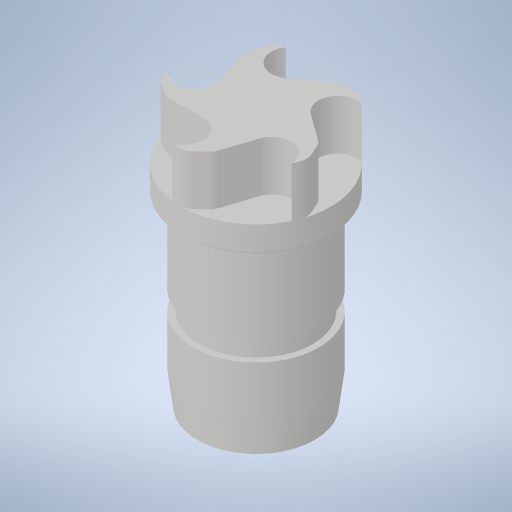
# Autodesk Inventor part: 3.2mm_uncorrected_thin
Saved by Autodesk Inventor 2023.1 (Build 271208000, 208)
## iProperties
Created: 2020-02-22
Part Number: 3.2mm_uncorrected_thin
Material: Generic
Document SubType Name: Modeling
Designer: kongooi
Density: 1 g/cm^3
Appearance: Default
Author: kongooi
Autodesk Inventor part; units mm, degrees
ref_plane "YZ Plane" through (0, 0, 0) normal (1, 0, 0) x (0, 1, 0)
sketch "Sketch2" plane through (0, 0, 0) normal (0, 1, 0) x (-1, 0, 0)
  line L0 (-0.3288, 1.3184) -> (-0.1582, 1.472)
  line L1 (-0.3288, 1.3184) -> (-0.1582, 1.472)
  line L2 (-0.5094, -1.2599) -> (-0.7376, -1.2837)
  arc A0 (0.7438, -1.3598) -> (0.1795, -0.809) centre (0.4146, -1.1327) ccw
  line L3 (-0.365, -1.2045) -> (0.1795, -0.809)
  arc A1 (-1.0634, -1.1277) -> (-0.954, -1.2216) centre (-0.0001, 0.0001) ccw
  line L4 (-0.365, -1.2045) -> (0.1795, -0.809)
  arc A2 (-0.5094, -1.2599) -> (-0.365, -1.2045) centre (-0.5404, -0.963) ccw
  line L5 (1.1525, 0.72) -> (1.3512, 0.6052)
  arc A3 (0.1974, 1.5374) -> (0.3303, 0.7602) centre (0.3304, 1.1602) ccw
  line L6 (1.0031, 0.7601) -> (0.3303, 0.7602)
  arc A4 (1.1525, 0.72) -> (1.0031, 0.7601) centre (1.0031, 0.4616) ccw
  line L7 (1.0407, -0.8744) -> (0.993, -1.0981)
  arc A5 (1.5231, 0.2873) -> (0.8243, -0.0783) centre (1.2047, 0.0452) ccw
  line L8 (1.0326, -0.7199) -> (0.8243, -0.0783)
  arc A6 (1.0407, -0.8744) -> (1.0326, -0.7199) centre (0.7487, -0.8121) ccw
  arc A7 (-1.4012, 0.663) -> (-0.621, 0.5492) centre (-1.0013, 0.6728) ccw
  line L9 (-0.413, 1.1889) -> (-0.621, 0.5492)
  arc A8 (-0.3288, 1.3184) -> (-0.413, 1.1889) centre (-0.1291, 1.0966) ccw
  line L10 (-1.3557, 0.0951) -> (-1.4489, 0.3047)
  arc A9 (-1.0634, -1.1277) -> (-0.7141, -0.4208) centre (-0.9492, -0.7444) ccw
  line L11 (-1.2585, -0.0252) -> (-0.7141, -0.4208)
  arc A10 (-1.3557, 0.0951) -> (-1.2585, -0.0252) centre (-1.083, 0.2163) ccw
  arc A11 (1.5231, 0.2872) -> (1.4898, 0.4277) centre (-0.0001, 0.0001) ccw
  arc A12 (-1.4012, 0.663) -> (-1.4567, 0.5298) centre (-0.0001, 0.0001) ccw
  arc A13 (0.7438, -1.3598) -> (0.867, -1.2847) centre (-0.0001, 0.0001) ccw
  arc A14 (0.1974, 1.5374) -> (0.0535, 1.5491) centre (-0.0001, 0.0001) ccw
  arc A15 (0.0535, 1.5491) -> (-0.1582, 1.472) centre (0.0431, 1.2484) ccw
  arc A16 (-1.4567, 0.5298) -> (-1.4489, 0.3047) centre (-1.174, 0.4269) ccw
  arc A17 (1.4898, 0.4277) -> (1.3512, 0.6052) centre (1.2005, 0.3447) ccw
  arc A18 (-0.954, -1.2216) -> (-0.7376, -1.2837) centre (-0.7688, -0.9844) ccw
  arc A19 (0.867, -1.2847) -> (0.993, -1.0981) centre (0.6987, -1.0353) ccw
  circle A20 centre (-0.0001, 0.0001) radius 1.55
  point P0 (-1.356, 0.0956)
  point P1 (1.0033, 0.76)
  point P2 (0.3301, 0.76)
  dimension "d305" = 3.1
  constraints: 49 point on circle, 26 tangent, 24 end point, 20 centre point, 12 equal radius, 2 coincident, 2 collinear, 3 other
sketch "Sketch3" plane through (0, 0, 0) normal (0, 1, 0) x (-1, 0, 0)
  line L0 (5.0133, 39.043) -> (38.6813, 7.297)
  line L1 (38.6813, 7.297) -> (18.893, -34.5332)
  line L2 (18.893, -34.5332) -> (-27.0048, -28.6397)
  line L3 (-27.0048, -28.6397) -> (-35.5829, 16.8329)
  line L4 (-35.5829, 16.8329) -> (5.0133, 39.043)
  circle A0 centre (0, 0) radius 39.3635
  circle A1 centre (0, 0) radius 20.4353
  circle A2 centre (0, 0) radius 31.8458
  circle A3 centre (10.4717, -28.7325) radius 10.093
  circle A4 centre (41.1153, -0.5956) radius 4.0726
  circle A5 centre (8.144, 29.3283) radius 10.0252
  circle A6 centre (-25.3778, 16.9956) radius 10.0583
  circle A7 centre (-24.1576, -18.872) radius 10.1582
  line L5 (-25.3778, 16.9956) -> (8.3216, 29.3877)
  line L6 (8.3216, 29.3877) -> (30.5209, 1.1669)
  line L7 (30.5209, 1.1669) -> (10.5413, -28.6665)
  line L8 (10.5413, -28.6665) -> (-24.006, -18.8838)
  line L9 (-24.006, -18.8838) -> (-25.3778, 16.9956)
  line L10 (-31.306, -23.8626) -> (-32.3687, 22.3998)
  line L11 (-32.3687, 22.3998) -> (11.301, 37.7064)
  line L12 (11.301, 37.7064) -> (39.3531, 0.904)
  line L13 (39.3531, 0.904) -> (13.0206, -37.1477)
  line L14 (13.0206, -37.1477) -> (-31.306, -23.8626)
  point P0 (-9.1427, -30.5051)
  constraints: 30 end point, 6 centre point, 6 coincident, 4 tangent, 1 midpoint, 43 other
extrude "Extrusion4" add sketch "Sketch2" against normal blind 1.032 contours L0 A15 A14 A3 L6 A4 L5 A17 A11 A5 L8 A6 L7 A19 A13 A0 L3 A2 L2 A18 A1 A9 L11 A10 L10 A16 A12 A7 L9 A8
sketch "Sketch6" plane through (0, -1.032, 0) normal (0, -1, 0) x (1, 0, 0)
  circle A0 centre (0, 0) radius 1.55
  dimension "d304" = 3.1
  constraints: 1 centre point, 1 coincident
  measures "d304" diameter of A0
extrude "Extrusion5" add sketch "Sketch6" along normal blind 0.55
ref_plane "Plan de construction1" through (0, -1.582, 0) normal (0, -1, 0) x (1, 0, 0)
sketch "Sketch7" plane through (0, -1.582, 0) normal (0, -1, 0) x (1, 0, 0)
  circle A0 centre (0, 0) radius 1.3
  circle A1 centre (0, 0) radius 0.6
  circle A2 centre (0, 0) radius 1.175
  dimension "d303" = 2.6
  dimension "d306" = 1.2
  dimension "d307" = 2.35
  constraints: 3 centre point, 2 coincident
  measures "d303" diameter of A0
  measures "d306" diameter of A1
  measures "d307" diameter of A2
extrude "Extrusion6" add sketch "Sketch7" along normal blind 3.8 contours A0 | A2
ref_plane "Plan de construction2" through (0, -3.282, 0) normal (0, -1, 0) x (1, 0, 0)
extrude "Extrusion7" cut sketch "Sketch7" along normal blind 0.4 from surface at 1.7 contours A0
chamfer "Chanfrein2" distance 0.7 angle 7 1 edges at (-1.3, -5.382, 0) measured on face at (1.2958, -4.8153, -0.1046)
chamfer "Chanfrein3" distance 0.05 angle 45 1 edges at (-1.55, -1.582, 0)
body "Solid4"
